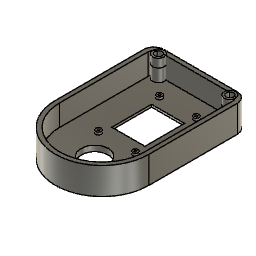
lime-display (Autodesk Fusion 360 archive; units mm, degrees)
design "lime-display.v01"
Autodesk Fusion 360 part; units mm, degrees
sketch "Dashboard Outline" plane through (0, 0, 0) normal (0, 0, 1) x (1, 0, 0)
  line L0 (-26, 102.2843) -> (26, 102.2843)
  line L1 (33, 95.2843) -> (33, 32.8067)
  line L2 (23.5263, 9.6655) -> (0, 9.6655)
  line L3 (-33, 32.8066) -> (-33, 95.2843)
  arc A0 (-33, 32.8066) -> (33, 32.8067) centre (0, 32.8066) ccw
  circle A1 centre (0, 27.5566) radius 9.525
  circle A2 centre (-13, 86.2843) radius 2
  circle A3 centre (13, 86.2843) radius 2
  circle A4 centre (13, 43.2843) radius 2
  circle A5 centre (-13, 43.2843) radius 2
  line L4 (0, 1.75) -> (0, 22.5)
  line L5 (-13.985, 81.6543) -> (13.985, 81.6543)
  line L6 (13.985, 81.6543) -> (13.985, 49.0243)
  line L7 (13.985, 49.0243) -> (-13.985, 49.0243)
  line L8 (-13.985, 49.0243) -> (-13.985, 81.6543)
  circle A6 centre (-13, 86.2843) radius 0.8
  circle A7 centre (13, 86.2843) radius 0.8
  circle A8 centre (-13, 43.2843) radius 0.8
  circle A9 centre (13, 43.2843) radius 0.8
  circle A10 centre (0, 27.5566) radius 13
  circle A11 centre (11.2625, 27.5566) radius 0.8
  circle A12 centre (-11.2625, 27.5566) radius 0.8
  line L9 (13, 27.5566) -> (9.525, 27.5566)
  line L10 (-9.525, 27.5566) -> (-13, 27.5566)
  circle A13 centre (-11.2625, 27.5566) radius 0.625
  circle A14 centre (11.2625, 27.5566) radius 0.625
  arc A15 (-26, 102.2843) -> (-33, 95.2843) centre (-26, 95.2843) ccw
  arc A16 (33, 95.2843) -> (26, 102.2843) centre (26, 95.2843) ccw
  circle A17 centre (-25.25, 97.7843) radius 2.5
  circle A18 centre (-25.25, 97.7843) radius 4
  circle A19 centre (25.25, 97.7843) radius 2.5
  circle A20 centre (25.25, 97.7843) radius 4
  dimension "d1" = 66
  dimension "d5" = 19.05
  dimension "d57" = 4
  dimension "d58" = 4
  dimension "d64" = 66
  dimension "d66" = 26
  dimension "d67" = 4
  dimension "d68" = 4
  dimension "d70" = 43
  dimension "d79" = 27.97
  dimension "d80" = 32.63
  dimension "d82" = 4.63
  dimension "d83" = 1.6
  dimension "d84" = 1.6
  dimension "d85" = 1.6
  dimension "d86" = 1.6
  dimension "d93" = 26
  dimension "d103" = 5.25
  dimension "d105" = 1.6
  dimension "d106" = 1.6
  dimension "d107" = 1.25
  dimension "d108" = 1.25
  dimension "d121" = 16
  dimension "d137" = 26
  dimension "d138" = 7
  dimension "d139" = 7
  dimension "d144" = 5
  dimension "d145" = 8
  dimension "d146" = 5
  dimension "d147" = 8
  dimension "d148" = 7.75
  dimension "d149" = 7.75
  dimension "d150" = 4.5
  dimension "d151" = 4.5
  constraint horizontal L0
  constraint vertical L1
  constraint horizontal L2
  constraint vertical L3
  constraint coincident A0 L2.start
  constraint symmetric A2 A3 L4
  constraint horizontal L5
  constraint vertical L6
  constraint horizontal L7
  constraint vertical L8
  constraint symmetric L4 L6 L8
  constraint concentric A2 A6
  constraint concentric A3 A7
  constraint concentric A5 A8
  constraint concentric A4 A9
  constraint concentric A1 A10
  constraint coincident A10 L9.start
  constraint coincident A10 L10.end
  constraint horizontal L9
  constraint coincident A1 L9.end
  constraint coincident A1 L10.start
  constraint collinear L9 L10
  constraint midpoint A11.centre L9
  constraint midpoint A12.centre L10
  constraint concentric A12 A13
  constraint concentric A11 A14
  constraint symmetric L4 A5.centre A4.centre
  constraint tangent L3 A15
  constraint tangent L0 A15
  constraint tangent L0 A16
  constraint tangent L1 A16
  constraint concentric A17 A18
  constraint concentric A19 A20
  measures "d1" diameter of A0
  measures "d5" diameter of A1
  measures "d57" diameter of A2
  measures "d58" diameter of A3
  measures "d64" distance of L1 L3
  measures "d66" distance of A2.centre A3.centre
  measures "d67" diameter of A5
  measures "d68" diameter of A4
  measures "d70" distance of A2.centre A5.centre
  measures "d79" distance of L5.start L5.end
  measures "d80" distance of L5.start L7.end
  measures "d82" distance of A2.centre L5
  measures "d83" diameter of A6
  measures "d84" diameter of A7
  measures "d85" diameter of A8
  measures "d86" diameter of A9
  measures "d93" diameter of A10
  measures "d103" distance of A0.centre A1.centre
  measures "d105" diameter of A11
  measures "d106" diameter of A12
  measures "d107" diameter of A13
  measures "d108" diameter of A14
  measures "d121" distance of L0 A2.centre
  measures "d137" distance of A5.centre A4.centre
  measures "d138" radius of A15
  measures "d139" radius of A16
  measures "d144" diameter of A17
  measures "d145" diameter of A18
  measures "d146" diameter of A19
  measures "d147" diameter of A20
  measures "d148" distance of L3 A17.centre
  measures "d149" distance of L1 A19.centre
  measures "d150" distance of L0 A17.centre
  measures "d151" distance of L0 A19.centre
extrude "Extrude3" add sketch "Dashboard Outline" along normal blind 4 contours L0 L1 L3 A0 A15 A16 | A1 L4 A10 A11 L9 | A1 A10 A11 A12 L9 L10 | A1 L4 A10 A12 L10 | A11 L9 A14 | A11 L9 A14 | A12 L10 A13 | A12 L10 A13 | L9 A14 | L9 A14 | L10 A13 | L10 A13 | A2 | A3 | A4 | A5 | A6 | A7 | A8 | A9 | A17 | A18 | A19 | A20 makes body 1
extrude "Extrude6" add sketch "Dashboard Outline" along normal blind 1.75 separate body contours A2 | A3 | A4 | A5 makes body 2 at (14.843, 87.0612, 1.1667) makes body 3 at (-11.0099, 43.0852, 1.1667) makes body 4 at (-14.843, 85.5074, 1.1667) makes body 5 at (14.9901, 43.0852, 1.1667)
move_body "Move2" bodies 3 2 5 4 to x (1, 0, 0) y (0, 1, 0) z (0, 0, 1) at (0, 0, 4)
move_face "MoveFace9" to x (0.866025, 0, -0.5) y (0, 1, 0) z (0.5, 0, 0.866025) at (-1.8736, 0, -6.9925) 1 faces at (-13.985, 59.901, 1.3333) on bodies 1
move_face "MoveFace10" to x (1, 0, 0) y (0, 0.866025, -0.5) z (0, 0.5, 0.866025) at (0, 6.568, 24.5122) 1 faces at (-3.8919, 49.0243, 1.3333) on bodies 1
move_face "MoveFace11" to x (0.866025, 0, 0.5) y (0, 1, 0) z (-0.5, 0, 0.866025) at (1.8736, 0, -6.9925) 1 faces at (13.985, 60.6708, 1.3333) on bodies 1
move_face "MoveFace12" to x (1, 0, 0) y (0, 0.866025, 0.5) z (0, -0.5, 0.866025) at (0, 10.9396, -40.8272) 1 faces at (3.8919, 81.6543, 1.3333) on bodies 1
extrude "Extrude7" add sketch "Dashboard Outline" along normal blind 1.75 contours A1 L4 A10 A11 L9 | A1 A10 A11 A12 L9 L10 | A1 L4 A10 A12 L10 | A11 L9 A14 | A11 L9 A14 | A12 L10 A13 | A12 L10 A13 | L9 A14 | L9 A14 | L10 A13 | L10 A13 bodies 1
extrude "Extrude8" add sketch "Dashboard Outline" along normal blind 1.75 contours A1 L4 A10 A11 L9 | A1 A10 A11 A12 L9 L10 | A1 L4 A10 A12 L10 | A11 L9 A14 | A11 L9 A14 | A12 L10 A13 | A12 L10 A13 | L9 A14 | L9 A14 | L10 A13 | L10 A13 bodies 1
extrude "Extrude9" add sketch "Dashboard Outline" along normal blind 1.75 separate body contours A1 L4 A10 A11 L9 | A1 A10 A11 A12 L9 L10 | A1 L4 A10 A12 L10 | A11 L9 A14 | A11 L9 A14 | A12 L10 A13 | A12 L10 A13 | L9 A14 | L9 A14 | L10 A13 | L10 A13 makes body 6
move_body "Move3" bodies 6 to x (1, 0, 0) y (0, 1, 0) z (0, 0, 1) at (0, 0, 4)
move_body "Move4" bodies 6 to x (1, 0, 0) y (0, 1, 0) z (0, 0, 1) at (0, 0, -5.75)
copy_body "Body->Comp1" bodies 6 removing the originals makes body 7 in component "Lock Raise Ring"
hole "Hole1" at (-11.2625, 27.2955, 0) direction (0, 0, 1) diameter 1.6 depth 1 tip angle 180 bodies 1
hole "Hole2" at (11.2625, 27.2955, 0) direction (0, 0, 1) diameter 1.6 depth 1 tip angle 180 bodies 1
extrude "Extrude10" add sketch "Dashboard Outline" along normal blind 1 separate body contours L9 A14 | L9 A14 | L10 A13 | L10 A13 makes body 8 at (11.6989, 27.1092, 0.6667) makes body 9 at (-10.6406, 27.6189, 0.6667)
combine "Combine1" operation add target body 7 tool bodies 8 9 in component "Lock Raise Ring"
combine "Combine1'" operation add target body 1 tool bodies 4 2 5 3
copy_body "Body->Comp7" bodies 1 removing the originals makes body 10 in component "dashboard-body-1"
move_face "MoveFace1" by (0, 0, -0.25) 2 faces at (-11.1275, 27.3716, 1) (11.3924, 27.2709, 1) on bodies 7 in component "Lock Raise Ring"
extrude "Extrude1" add sketch "Dashboard Outline" along normal blind 2 separate body contours L5 L6 L7 L8 makes body 11 in component "lens"
move_face "MoveFace1'" to x (1, 0, 0) y (0, 0.866025, 0.5) z (0, -0.5, 0.866025) at (0, 10.9396, -40.8272) 1 faces at (-4.6617, 81.6543, 0.6667) on bodies 11 in component "lens"
move_face "MoveFace2" to x (0.866025, 0, 0.5) y (0, 1, 0) z (-0.5, 0, 0.866025) at (1.8736, 0, -6.9925) 1 faces at (13.985, 70.3927, 0.6667) on bodies 11 in component "lens"
move_face "MoveFace3" to x (1, 0, 0) y (0, 0.866025, -0.5) z (0, 0.5, 0.866025) at (0, 6.568, 24.5122) 1 faces at (4.2768, 49.0243, 0.6667) on bodies 11 in component "lens"
move_face "MoveFace4" to x (0.866025, 0, -0.5) y (0, 1, 0) z (0.5, 0, 0.866025) at (-1.8736, 0, -6.9925) 1 faces at (-13.985, 70.3927, 0.6667) on bodies 11 in component "lens"
extrude "Extrude11" add sketch "Dashboard Outline" along normal blind 19 thin wall 3 on the right separate body open curves A16 L1 A0 L3 A15 L0 makes body 12
combine "Combine1''" operation add target body 10 tool bodies 12 keep tools in component "dashboard-body-1"
move_face "OffsetFaces1" offset -0.25 1 faces at (-4.6617, 70.7776, 0) on bodies 11 in component "lens"
extrude "Extrude12" add sketch "Dashboard Outline" along normal blind 9 separate body contours A17 | A18 makes body 13
extrude "Extrude13" add sketch "Dashboard Outline" along normal blind 9 separate body contours A19 | A20 makes body 14
extrude "Extrude14" add sketch "Dashboard Outline" along normal blind 6 separate body contours A20 makes body 15
move_body "Move5" bodies 15 to x (1, 0, 0) y (0, 1, 0) z (0, 0, 1) at (0, 0, 9)
move_body "Move6" bodies 14 to x (1, 0, 0) y (0, 1, 0) z (0, 0, 1) at (0, 0, 4)
move_body "Move7" bodies 15 to x (1, 0, 0) y (0, 1, 0) z (0, 0, 1) at (0, 0, 4)
move_body "Move8" bodies 13 to x (1, 0, 0) y (0, 1, 0) z (0, 0, 1) at (0, 0, 4)
extrude "Extrude15" add sketch "Dashboard Outline" along normal blind 6 separate body contours A18 makes body 16
move_body "Move9" bodies 16 to x (1, 0, 0) y (0, 1, 0) z (0, 0, 1) at (0, 0, 13)
copy_body "CutPasteBodies1" bodies 12 removing the originals makes body 17 in component "dashboard-body-1"
copy_body "CutPasteBodies2" bodies 13 removing the originals makes body 18 in component "dashboard-body-1"
copy_body "CutPasteBodies3" bodies 14 removing the originals makes body 19 in component "dashboard-body-1"
copy_body "CutPasteBodies4" bodies 15 removing the originals makes body 20 in component "dashboard-body-1"
copy_body "CutPasteBodies5" bodies 16 removing the originals makes body 21 in component "dashboard-body-1"
delete_body "RemoveBody1" bodies 17 in component "dashboard-body-1"
hole "Hole1'" at (-25.25, 97.7843, 19) direction (0, 0, -1) diameter 5 depth 6 tip angle 180 bodies 10 in component "dashboard-body-1"
hole "Hole2'" at (25.25, 97.7843, 19) direction (0, 0, -1) diameter 5 depth 6 tip angle 180 bodies 10 in component "dashboard-body-1"
component "lens" placed x (1, 0, 0) y (0, 1, 0) z (0, 0, 1) at (0, 0, 0)
component "Lock Raise Ring" placed x (1, 0, 0) y (0, 1, 0) z (0, 0, 1) at (0, 0, 0)
component "dashboard-body-1" placed x (1, 0, 0) y (0, 1, 0) z (0, 0, 1) at (0, 0, 0)
named bodies: "dashboard-body-1", "screen-mount2", "screen-mount4", "screen-mount1", "screen-mount3", "Lock Raise Ring", "dashboard-body-plate", "main-extrusion", "top-right-attachment-base", "top-left-attachment-base", "top-left-attachment-thread-receiver", "top-right-attachment-thread-receiver"
